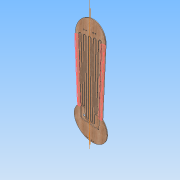
# Autodesk Inventor part: HOT Ply back
Saved by Autodesk Inventor 2013 (Build 170138000, 138)
## iProperties
Created: 2018-07-29
Part Number: HOT Ply back
Material: Wood (Birch)
Document SubType Name: Modeling
Designer: Jeff Vyduna
Density: 1 g/cm^3
Author: Jeff Vyduna
Autodesk Inventor part; units mm, degrees
ref_plane "YZ Plane" through (0, 0, 0) normal (1, 0, 0) x (0, 1, 0)
ref_plane "XZ Plane" through (0, 0, 0) normal (0, 1, 0) x (-1, 0, 0)
ref_plane "XY Plane" through (0, 0, 0) normal (0, 0, 1) x (1, 0, 0)
sketch "One rope curve" plane through (0, 0, 0) normal (0, 0, 1) x (1, 0, 0)
  arc A0 (29.7678, 76.5416) -> (92.7598, 76.5416) centre (61.2638, 76.5416) ccw
  arc A1 (41.9598, 76.5416) -> (80.5678, 76.5416) centre (61.2638, 76.5416) ccw
  line L0 (29.7678, 1397.3416) -> (29.7678, 76.5416)
  line L1 (41.9598, 1397.3416) -> (41.9598, 76.5416)
  line L2 (80.5678, 76.5416) -> (80.5678, 1397.3416)
  line L3 (92.7598, 76.5416) -> (92.7598, 1397.3416)
  arc A2 (29.7678, 1397.3416) -> (-8.8402, 1397.3416) centre (10.4638, 1397.3416) ccw
  arc A3 (41.9598, 1397.3416) -> (-21.0322, 1397.3416) centre (10.4638, 1397.3416) ccw
  dimension "d31" = 1320.8
  dimension "d32" = 31.496
  dimension "d33" = 31.496
  dimension "d34" = 12.192
  measures "d31" vertical distance of A1.centre A2.centre
  measures "d32" radius of A3
  measures "d33" radius of A0
  measures "d34" distance of A3.end A2.end
sketch "Cut thermo stock" plane through (0, 0, 0) normal (0, 0, 1) x (1, 0, 0)
  line L0 (304.8, 305.8565) -> (304.8, 1689.1)
  line L1 (-304.8, 1689.1) -> (-304.8, 305.8565)
  arc A0 (304.8, 1689.1) -> (-304.8, 1689.1) centre (0, 1689.1) ccw
  arc A1 (-304.8, 305.8565) -> (304.8, 305.8565) centre (0, 0) ccw
  line L2 (0, 1993.9) -> (0, -431.8)
  dimension "d0" = 2425.7
  dimension "d2" = 431.8
  dimension "d3" = 304.8
  constraints: 6 end point, 6 point on circle, 2 centre point, 2 line through centre, 2 parallel, 2 point on line, 2 tangent, 1 coincident, 1 vertical
  measures "d0" distance of L2.start L2.end
  measures "d2" radius of A1
  measures "d3" radius of A0
extrude "Extrusion1" add sketch "Cut thermo stock" along normal blind 18.034
sketch "Hole Sketch" plane through (0, 0, 18.034) normal (0, 0, 1) x (1, 0, 0)
  arc A0 (304.8, 1689.1) -> (-304.8, 1689.1) centre (0, 1689.1) ccw projected
  arc A1 (-304.8, 305.8565) -> (304.8, 305.8565) centre (0, 0) ccw projected
  arc A2 (304.8, 1689.1) -> (-304.8, 1689.1) centre (0, 1689.1) ccw projected
  line L0 (-304.8, 1689.1) -> (-304.8, 305.8565) projected
  arc A3 (-304.8, 305.8565) -> (304.8, 305.8565) centre (0, 0) ccw projected
  line L1 (304.8, 305.8565) -> (304.8, 1689.1) projected
  point P0 (-96.8375, -384.8795)
  point P1 (50.8, -384.8795)
  point P2 (96.8375, -384.8795)
  point P3 (-50.8, -384.8795)
  point P4 (-69.85, 1799.5205)
  point P5 (-115.8875, 1799.5205)
  point P6 (69.85, 1799.5205)
  point P7 (115.8875, 1799.5205)
  dimension "uBoltSpacing" = 46.0375
  dimension "d8" = 46.0375
  dimension "d9" = 101.6
  dimension "d10" = 46.0375
  dimension "d11" = 46.0375
  dimension "d12" = 19.05
  dimension "d13" = 19.05
  dimension "d14" = 50.8
  dimension "d15" = 396.875
  dimension "d16" = 160.0706
  dimension "d17" = 2184.4
  constraints: 6 horizontal alignment
  measures "uBoltSpacing" distance of point (-50.8, -384.88) point (-96.838, -384.88)
  measures "d8" distance of point (96.838, -384.88) point (50.8, -384.88)
  measures "d9" distance of point (50.8, -384.88) point (-50.8, -384.88)
  measures "d10" distance of point (-115.888, 1799.52) point (-69.85, 1799.52)
  measures "d11" distance of point (115.888, 1799.52) point (69.85, 1799.52)
  measures "d12" horizontal distance of point (69.85, 1799.52) point (50.8, -384.88)
  measures "d13" horizontal distance of point (-50.8, -384.88) point (-69.85, 1799.52)
  measures "d14" horizontal distance of point (50.8, -384.88) A1.centre
  measures "d15" distance of point (96.838, -384.88) A1.centre
  measures "d16" distance of point (115.888, 1799.52) A0.centre
  measures "d17" vertical distance of point (96.838, -384.88) point (69.85, 1799.52)
ref_plane "Work Plane1" through (0, 305.8565, 0) normal (1, 0, 0) x (0, 0, -1)
hole "Hole1" at (-96.8375, -384.8795, 18.034) at (50.8, -384.8795, 18.034) at (96.8375, -384.8795, 18.034) at (-50.8, -384.8795, 18.034) at (-69.85, 1799.5205, 18.034) at (-115.8875, 1799.5205, 18.034) at (69.85, 1799.5205, 18.034) at (115.8875, 1799.5205, 18.034) direction (0, 0, -1) diameter 9.525 end through all counterbore diameter 19.05 counterbore depth 6.35
sketch "Sketch3" plane through (0, 0, 18.034) normal (0, 0, 1) x (1, 0, 0)
  arc A0 (304.8, 1689.1) -> (-304.8, 1689.1) centre (0, 1689.1) ccw projected
  line L0 (-304.8, 1689.1) -> (-304.8, 305.8565) projected
  arc A1 (-304.8, 305.8565) -> (304.8, 305.8565) centre (0, 0) ccw projected
  line L1 (-241.3, 1689.1) -> (-241.3, 305.8565) construction
  line L2 (0, 0) -> (0, 1689.1) construction
  line L3 (241.3, 1689.1) -> (241.3, 305.8565) construction
  line L4 (0, 13.7565) -> (-209.296, 13.7565)
  line L5 (-234.696, 39.1565) -> (-234.696, 1702.8565)
  line L6 (-222.504, 356.6565) -> (-222.504, 1702.8565)
  arc A2 (222.504, 1702.8565) -> (183.896, 1702.8565) centre (203.2, 1702.8565) ccw
  arc A3 (234.696, 1702.8565) -> (171.704, 1702.8565) centre (203.2, 1702.8565) ccw
  arc A4 (-222.504, 356.6565) -> (-197.104, 331.2565) centre (-197.104, 356.6565) ccw
  arc A5 (-234.696, 39.1565) -> (-209.296, 13.7565) centre (-209.296, 39.1565) ccw
  line L7 (0, 13.7565) -> (209.296, 13.7565)
  line L8 (234.696, 39.1565) -> (234.696, 1702.8565)
  line L9 (222.504, 356.6565) -> (222.504, 1702.8565)
  arc A6 (197.104, 331.2565) -> (222.504, 356.6565) centre (197.104, 356.6565) ccw
  arc A7 (209.296, 13.7565) -> (234.696, 39.1565) centre (209.296, 39.1565) ccw
  arc A8 (-171.704, 1702.8565) -> (-234.696, 1702.8565) centre (-203.2, 1702.8565) ccw
  arc A9 (-183.896, 1702.8565) -> (-222.504, 1702.8565) centre (-203.2, 1702.8565) ccw
  line L10 (-183.896, 1702.8565) -> (-183.896, 382.0565)
  line L11 (-171.704, 1702.8565) -> (-171.704, 382.0565)
  arc A10 (-171.704, 382.0565) -> (-133.096, 382.0565) centre (-152.4, 382.0565) ccw
  arc A11 (-183.896, 382.0565) -> (-120.904, 382.0565) centre (-152.4, 382.0565) ccw
  line L12 (-133.096, 382.0565) -> (-133.096, 1702.8565)
  line L13 (-120.904, 382.0565) -> (-120.904, 1702.8565)
  arc A12 (-70.104, 1702.8565) -> (-133.096, 1702.8565) centre (-101.6, 1702.8565) ccw
  arc A13 (-82.296, 1702.8565) -> (-120.904, 1702.8565) centre (-101.6, 1702.8565) ccw
  line L14 (-82.296, 1702.8565) -> (-82.296, 128.0565)
  line L15 (-70.104, 1702.8565) -> (-70.104, 128.0565)
  arc A14 (-70.104, 128.0565) -> (-31.496, 128.0565) centre (-50.8, 128.0565) ccw
  arc A15 (-82.296, 128.0565) -> (-19.304, 128.0565) centre (-50.8, 128.0565) ccw
  line L16 (-31.496, 128.0565) -> (-31.496, 1702.8565)
  line L17 (-19.304, 128.0565) -> (-19.304, 1702.8565)
  arc A16 (31.496, 1702.8565) -> (-31.496, 1702.8565) centre (0, 1702.8565) ccw
  arc A17 (19.304, 1702.8565) -> (-19.304, 1702.8565) centre (0, 1702.8565) ccw
  line L18 (19.304, 1702.8565) -> (19.304, 128.0565)
  line L19 (31.496, 1702.8565) -> (31.496, 128.0565)
  arc A18 (31.496, 128.0565) -> (70.104, 128.0565) centre (50.8, 128.0565) ccw
  arc A19 (19.304, 128.0565) -> (82.296, 128.0565) centre (50.8, 128.0565) ccw
  line L20 (70.104, 128.0565) -> (70.104, 1702.8565)
  line L21 (82.296, 128.0565) -> (82.296, 1702.848)
  arc A20 (133.096, 1702.8565) -> (70.104, 1702.8565) centre (101.6, 1702.8565) ccw
  arc A21 (120.904, 1702.8565) -> (82.296, 1702.848) centre (101.6, 1702.8565) ccw
  line L22 (120.904, 1702.8565) -> (120.904, 382.0565)
  line L23 (133.096, 1702.8565) -> (133.096, 382.0565)
  arc A22 (133.096, 382.0565) -> (171.704, 382.0565) centre (152.4, 382.0565) ccw
  arc A23 (120.904, 382.0565) -> (183.896, 382.0565) centre (152.4, 382.0565) ccw
  line L24 (171.704, 382.0565) -> (171.704, 1702.8565)
  line L25 (183.896, 382.0565) -> (183.896, 1702.8565)
  line L26 (276.8918, -213.6858) -> (267.2398, -206.237) projected
  arc A24 (276.8918, -213.6858) -> (241.3, 253.1896) centre (0, 0) ccw projected
  line L27 (241.3, 236.0617) -> (241.3, 253.1896) projected
  arc A25 (267.2398, -206.237) -> (241.3, 236.0617) centre (0, 0) ccw projected
  line L28 (-322.1355, -248.6018) -> (-331.7875, -256.0505) projected
  arc A26 (-293.9585, 281.3583) -> (-322.1355, -248.6018) centre (0, 0) ccw projected
  arc A27 (-280.0129, 287.3145) -> (-293.9585, 281.3583) centre (-280.0129, 268.0105) ccw projected
  line L29 (-253.6042, 287.3145) -> (-280.0129, 287.3145) projected
  arc A28 (-239.1182, 255.2512) -> (-253.6042, 287.3145) centre (-253.6042, 268.0105) ccw projected
  arc A29 (-239.1182, 255.2512) -> (-276.8918, -213.6858) centre (0, 0) ccw projected
  line L30 (-267.2398, -206.237) -> (-276.8918, -213.6858) projected
  arc A30 (-230.7829, 246.3535) -> (-267.2398, -206.237) centre (0, 0) ccw projected
  arc A31 (-230.7829, 246.3535) -> (-253.6515, 299.5065) centre (-253.6515, 268.0105) ccw projected
  line L31 (-280.0129, 299.5065) -> (-253.6515, 299.5065) projected
  arc A32 (-280.0129, 299.5065) -> (-302.7663, 289.7886) centre (-280.0129, 268.0105) ccw projected
  arc A33 (-302.7663, 289.7886) -> (-331.7875, -256.0505) centre (0, 0) ccw projected
  arc A34 (-230.7829, 246.3535) -> (-267.2398, -206.237) centre (0, 0) ccw projected
  line L32 (-267.2398, -206.237) -> (-241.3, -186.2186) projected
  arc A35 (-196.85, 232.7082) -> (-241.3, -186.2186) centre (0, 0) ccw projected
  line L33 (-196.85, 232.7082) -> (-196.85, 305.8565) projected
  line L34 (-196.85, 305.8565) -> (-304.8, 305.8565) projected
  arc A36 (-304.8, 305.8565) -> (-341.8417, -263.8096) centre (0, 0) ccw projected
  line L35 (-341.8417, -263.8096) -> (-331.7875, -256.0505) projected
  arc A37 (-302.7663, 289.7886) -> (-331.7875, -256.0505) centre (0, 0) ccw projected
  arc A38 (-280.0129, 299.5065) -> (-302.7663, 289.7886) centre (-280.0129, 268.0105) ccw projected
  line L36 (-280.0129, 299.5065) -> (-253.6515, 299.5065) projected
  arc A39 (-230.7829, 246.3535) -> (-253.6515, 299.5065) centre (-253.6515, 268.0105) ccw projected
  line L37 (304.8, 305.8565) -> (304.8, 1689.1) projected
  line L38 (-120.904, 305.8565) -> (-120.904, 102.6565)
  line L39 (-95.504, 77.2565) -> (95.504, 77.2565)
  line L40 (120.904, 102.6565) -> (120.904, 305.8565)
  line L41 (-19.304, 331.2565) -> (0, 331.2565)
  line L42 (-197.104, 331.2565) -> (-146.304, 331.2565)
  line L43 (197.104, 331.2565) -> (146.304, 331.2565)
  arc A40 (-120.904, 305.8565) -> (-146.304, 331.2565) centre (-146.304, 305.8565) ccw
  arc A41 (146.304, 331.2565) -> (120.904, 305.8565) centre (146.304, 305.8565) ccw
  arc A42 (95.504, 77.2565) -> (120.904, 102.6565) centre (95.504, 102.6565) ccw
  arc A43 (-120.904, 102.6565) -> (-95.504, 77.2565) centre (-95.504, 102.6565) ccw
  point P0 (-120.904, 331.2565)
  point P1 (-120.904, 77.2565)
  point P2 (120.904, 77.2565)
  point P3 (120.904, 331.2565)
  dimension "d37" = 63.5
  dimension "d39" = 25.4
  dimension "d40" = 25.4
  dimension "d43" = 1320.8
  dimension "d44" = 31.496
  dimension "d45" = 31.496
  dimension "d46" = 12.192
  dimension "d50" = 1574.8
  dimension "d51" = 31.496
  dimension "d52" = 31.496
  dimension "d53" = 12.192
  dimension "d57" = 1574.8
  dimension "d58" = 31.496
  dimension "d59" = 31.496
  dimension "d64" = 1320.8
  dimension "d65" = 31.496
  dimension "d66" = 31.496
  dimension "d67" = 12.192
  dimension "d74" = 50.8
  dimension "d75" = 50.8
  dimension "d76" = 25.4
  dimension "d77" = 63.5
  dimension "d78" = 25.4
  constraints: 62 end point, 52 point on circle, 41 horizontal alignment, 29 tangent, 26 centre point, 20 parallel, 11 point on line, 10 symmetric about line, 9 concentric, 4 equal radius, 3 horizontal, 2 collinear, 1 perpendicular, 1 vertical, 2 other
  measures "d37" distance of L1.end L0.end
  measures "d39" radius of A4
  measures "d40" radius of A5
  measures "d43" vertical distance of A10.centre A9.centre
  measures "d44" radius of A8
  measures "d45" radius of A11
  measures "d46" distance of L5.end L6.end
  measures "d50" vertical distance of A14.centre A13.centre
  measures "d51" radius of A12
  measures "d52" radius of A15
  measures "d53" distance of L12.end L13.end
  measures "d57" vertical distance of A18.centre A17.centre
  measures "d58" radius of A16
  measures "d59" radius of A19
  measures "d64" vertical distance of A22.centre A21.centre
  measures "d65" radius of A20
  measures "d66" radius of A23
  measures "d67" distance of L20.end L21.end
  measures "d74" distance from line of L39 A14.centre
  measures "d75" distance from line of L42 A10.centre
  measures "d76" distance from line of L33.end L42
  measures "d77" distance between parallel lines of L39 L4
  measures "d78" radius of A40
extrude "Extrusion2" cut sketch "Sketch3" against normal blind 12.7 contours L34 L33 A35 L5 A30 A31 | L5 A8 L11 A10 L12 A12 L15 A14 L16 A16 L19 A18 L20 A20 L23 A22 L24 A3 L8 A7 L7 L4 A5 A35 L33 L34 | A31 A30 L5 A28 | A28 L5
sketch "Sketch4" plane through (0, 0, 5.334) normal (0, 0, 1) x (1, 0, 0)
  line L0 (-174.879, 147.1065) -> (-127.254, 147.1065)
  line L1 (-122.4915, 142.344) -> (-122.4915, 107.419)
  line L2 (-127.254, 102.6565) -> (-174.879, 102.6565)
  line L3 (-179.6415, 107.419) -> (-179.6415, 142.344)
  arc A0 (-174.879, 147.1065) -> (-179.6415, 142.344) centre (-174.879, 142.344) ccw
  arc A1 (-122.4915, 142.344) -> (-127.254, 147.1065) centre (-127.254, 142.344) ccw
  arc A2 (-127.254, 102.6565) -> (-122.4915, 107.419) centre (-127.254, 107.419) ccw
  arc A3 (-179.6415, 107.419) -> (-174.879, 102.6565) centre (-174.879, 107.419) ccw
  line L4 (-120.904, 305.8565) -> (-120.904, 102.6565) projected
  point P0 (0, 0)
  point P1 (-122.4915, 102.6565)
  point P2 (-122.4915, 147.1065)
  point P3 (-179.6415, 102.6565)
  dimension "d79" = 57.15
  dimension "d80" = 44.45
  dimension "d81" = 4.7625
  dimension "d84" = 1.5875
  constraints: 8 end point, 8 point on circle, 8 tangent, 6 point on line, 4 centre point, 3 equal radius, 2 parallel, 1 horizontal, 1 horizontal alignment, 1 perpendicular
  measures "d79" distance of point (-122.492, 102.657) point (-179.642, 102.657)
  measures "d80" distance of point (-122.492, 147.107) point (-122.492, 102.657)
  measures "d81" radius of A0
  measures "d84" distance between parallel lines of L4 L1
extrude "Through Hole" cut sketch "Sketch4" against normal through all
equation "\"d8\" = uBoltSpacing"
equation "\"d10\" = uBoltSpacing"
equation "\"d11\" = uBoltSpacing"
equation "\"d13\" = d12"
equation "\"d14\" = 0.5 * d9"
equation "\"d31\" = litH"
equation "\"d32\" = minBendR + 0.5 * bRopeChannel"
equation "\"d33\" = d32"
equation "\"d34\" = bRopeChannel"
equation "\"d39\" = minBendR"
equation "\"d40\" = minBendR"
equation "\"d43\" = d47"
equation "\"d44\" = d49 + 0.5 * d48"
equation "\"d45\" = d44"
equation "\"d46\" = d48"
equation "\"d51\" = d56 + 0.5 * d55"
equation "\"d52\" = d51"
equation "\"d53\" = d55"
equation "\"d58\" = d63 + 0.5 * d62"
equation "\"d59\" = d58"
equation "\"d64\" = d68"
equation "\"d65\" = d70 + 0.5 * d69"
equation "\"d66\" = d65"
equation "\"d67\" = d69"
equation "\"minBendR\" = 25.4"
equation "\"bRopeChannel\" = 12.192"
equation "\"litH\" = 1320.8"
equation "\"d47\" = 1320.8"
equation "\"d48\" = 12.192"
equation "\"d49\" = 25.4"
equation "\"d54\" = 1320.8"
equation "\"d55\" = 12.192"
equation "\"d56\" = 25.4"
equation "\"d61\" = 1320.8"
equation "\"d62\" = 12.192"
equation "\"d63\" = 25.4"
equation "\"d68\" = 1320.8"
equation "\"d69\" = 12.192"
equation "\"d70\" = 25.4"
body "Solid1"
